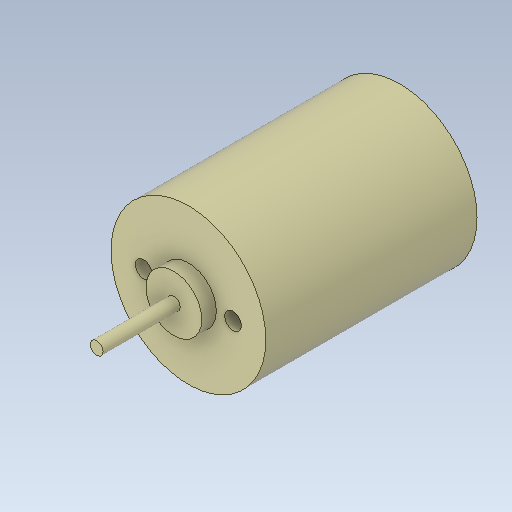
# Autodesk Inventor part: マブチモーター　RS-380PH
Saved by Autodesk Inventor 2020.2 (Build 242310000, 310)
## iProperties
Created: 2016-01-15
Part Number: マブチモーター　RS-380PH
Material: 一般
Document SubType Name: Modeling
Designer: Takumi
Density: 3.24274 g/cm^3
Appearance: 滑らか - 灰色
Mass: 75 g
Surface Area: 49.1237 cm^2
Volume: 23.1286 cm^3
Author: Takumi
Autodesk Inventor part; units mm, degrees
ref_plane "YZ Plane" through (0, 0, 0) normal (1, 0, 0) x (0, 1, 0)
ref_plane "XZ Plane" through (0, 0, 0) normal (0, 1, 0) x (-1, 0, 0)
ref_plane "XY Plane" through (0, 0, 0) normal (0, 0, 1) x (1, 0, 0)
sketch "スケッチ1" plane through (0, 0, 0) normal (0, 0, 1) x (1, 0, 0)
  circle A0 centre (0, 0) radius 13.85
  dimension "d0" = 27.7
  constraints: 1 centre point, 1 coincident
  measures "d0" diameter of A0
extrude "押し出し1" add sketch "スケッチ1" along normal blind 37.8
sketch "スケッチ2" plane through (0, 0, 37.8) normal (0, 0, 1) x (1, 0, 0)
  circle A0 centre (0, 0) radius 5
  dimension "d3" = 10
  constraints: 1 centre point, 1 coincident
  measures "d3" diameter of A0
extrude "押し出し2" add sketch "スケッチ2" along normal blind 2.6
sketch "スケッチ3" plane through (0, 0, 40.4) normal (0, 0, 1) x (1, 0, 0)
  circle A0 centre (0, 0) radius 1.15
  dimension "d6" = 2.3
  constraints: 1 centre point, 1 coincident
  measures "d6" diameter of A0
extrude "押し出し3" add sketch "スケッチ3" along normal blind 13.8
sketch "スケッチ4" plane through (0, 0, 0) normal (0, 0, -1) x (-1, 0, 0)
  circle A0 centre (0, 0) radius 1.15 projected
  circle A1 centre (0, 0) radius 5
  dimension "d9" = 10
  constraints: 1 centre point, 1 coincident
  measures "d9" diameter of A1
extrude "押し出し4" add sketch "スケッチ4" along normal blind 2.6
extrude "押し出し5" add sketch "スケッチ4" along normal blind 2.8 contours A0
sketch "スケッチ5" plane through (0, 0, 37.8) normal (0, 0, 1) x (1, 0, 0)
  circle A0 centre (-8, 0) radius 1.3
  circle A1 centre (8, 0) radius 1.3
  line L0 (-8, 0) -> (8, 0)
  point P0 (0, 0)
  point P1 (0, 0)
  dimension "d14" = 2.6
  dimension "d15" = 2.6
  dimension "d16" = 16
  dimension "d17" = 8
  constraints: 2 centre point, 2 end point, 1 coincident, 1 horizontal, 1 midpoint
  measures "d14" diameter of A0
  measures "d15" diameter of A1
  measures "d16" distance of L0.start L0.end
  measures "d17" distance of L0.start point (0, 0)
hole "穴1" at (-8, 0, 37.8) at (8, 0, 37.8) direction (0, 0, -1) diameter 3 depth 8 tip angle 118
